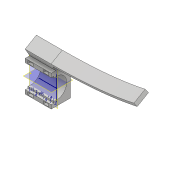
# Autodesk Inventor part: abrazadera_leds
Saved by Autodesk Inventor 2018 (Build 220112000, 112)
## iProperties
Created: 2018-08-01
Part Number: abrazadera_leds
Material: Generic
Document SubType Name: Sheet Metal
Designer: Bardo91
Density: 1 g/cm^3
Sheet Metal Rule: Default_mm
Appearance: Default
Author: Bardo91
Autodesk Inventor part; units mm, degrees
ref_plane "YZ Plane" through (0, 0, 0) normal (1, 0, 0) x (0, 1, 0)
ref_plane "XZ Plane" through (0, 0, 0) normal (0, 1, 0) x (-1, 0, 0)
ref_plane "XY Plane" through (0, 0, 0) normal (0, 0, 1) x (1, 0, 0)
sketch "Sketch1" plane through (0, 0, 0) normal (1, 0, 0) x (0, 1, 0)
  arc A0 (-2, -7.746) -> (-2, 7.746) centre (0, 0) ccw
  line L0 (0, 0) -> (-2, 0)
  line L1 (-2, 7.746) -> (-2, 9)
  line L2 (-2, 9) -> (-4, 9)
  line L3 (-4, 9) -> (-4, 12)
  line L4 (-4, 12) -> (11, 12)
  line L5 (-2, 0) -> (-2, -9)
  line L6 (-2, -9) -> (-4, -9)
  line L7 (-4, -9) -> (-4, -12)
  line L8 (-4, -12) -> (11, -12)
  line L9 (11, -12) -> (11, 12)
  line L10 (11, 12) -> (6, 20.6603)
  line L11 (11, 12) -> (21, 12) construction
  line L12 (6, 20.6603) -> (-2.6603, 15.6603)
  line L13 (-2.6603, 15.6603) -> (-0.547, 12)
  dimension "d0" = 16
  dimension "d1" = 2
  dimension "d2" = 9
  dimension "d3" = 2
  dimension "d4" = 3
  dimension "d5" = 15
  dimension "d6" = 9
  dimension "d7" = 3
  dimension "d8" = 10
  dimension "d9" = 120
  dimension "d10" = 10
  constraints: 28 end point, 9 perpendicular, 3 horizontal, 2 point on circle, 2 point on line, 1 centre point, 1 coincident, 1 equal length, 1 vertical
  measures "d0" diameter of A0
  measures "d1" distance of L0.start L0.end
  measures "d2" distance of L0.end L1.end
  measures "d3" distance of L1.end L2.end
  measures "d4" distance of L2.end L3.end
  measures "d5" distance of L3.end L4.end
  measures "d6" distance of L0.end L5.end
  measures "d7" distance of L6.end L7.end
  measures "d8" distance of L4.end L10.end
  measures "d9" angle of L11 L10
  measures "d10" distance of L10.end L12.end
extrude "Extrusion1" add sketch "Sketch1" along normal blind 20
ref_plane "Work Plane1" through (20, 8, 0) normal (0, 0, -1) x (-1, 0, 0)
ref_plane "Work Plane2" through (0, 0, 12) normal (0, 1, 0) x (1, 0, 0)
sketch "Sketch3" plane through (0, 0, 12) normal (0, 1, 0) x (1, 0, 0)
  line L0 (0, 21) -> (20, 21) projected
  line L1 (10, 21) -> (10, 22.5)
  line L2 (10, 22.5) -> (14, 22.5)
  line L3 (14, 22.5) -> (14, 21.5)
  line L4 (14, 21.5) -> (18, 21.5)
  line L5 (18, 21.5) -> (18, 23.5)
  line L6 (18, 23.5) -> (14, 23.5)
  line L7 (14, 23.5) -> (14, 22.5)
  line L8 (10, 22.5) -> (6, 22.5)
  line L9 (6, 22.5) -> (6, 23.5)
  line L10 (6, 23.5) -> (2, 23.5)
  line L11 (2, 23.5) -> (2, 21.5)
  line L12 (2, 21.5) -> (6, 21.5)
  line L13 (6, 22.5) -> (6, 21.5)
  line L14 (0, 3) -> (20, 3) projected
  line L15 (20, 21) -> (20, 3)
  line L16 (20, 20) -> (20, 4) projected
  line L17 (20, 12) -> (6.2446, 12)
  line L18 (0, 3) -> (20, 3)
  line L19 (10, 3) -> (10, 1.5)
  line L20 (10, 1.5) -> (14, 1.5)
  line L21 (14, 1.5) -> (14, 2.5)
  line L22 (14, 2.5) -> (18, 2.5)
  line L23 (18, 2.5) -> (18, 0.5)
  line L24 (18, 0.5) -> (14, 0.5)
  line L25 (14, 0.5) -> (14, 1.5)
  line L26 (10, 1.5) -> (6, 1.5)
  line L27 (6, 1.5) -> (6, 0.5)
  line L28 (6, 0.5) -> (2, 0.5)
  line L29 (2, 0.5) -> (2, 2.5)
  line L30 (2, 2.5) -> (6, 2.5)
  line L31 (6, 1.5) -> (6, 2.5)
  point P0 (0, 12)
  point P1 (20, 4.254)
  point P2 (20, 19.746)
  dimension "d25" = 1.5
  dimension "d26" = 4
  dimension "d27" = 1
  dimension "d28" = 4
  dimension "d29" = 2
  dimension "d30" = 4
  dimension "d31" = 1
  dimension "d32" = 4
  dimension "d33" = 2
  constraints: 58 end point, 14 point on line, 12 symmetric about line, 6 perpendicular, 2 horizontal, 2 midpoint, 1 vertical
  measures "d25" distance of L1.start L1.end
  measures "d26" distance of L1.end L2.end
  measures "d27" distance of L2.end L3.end
  measures "d28" distance of L3.end L4.end
  measures "d29" distance of L4.end L5.end
  measures "d30" distance of L1.end L8.end
  measures "d31" distance of L8.end L9.end
  measures "d32" distance of L9.end L10.end
  measures "d33" distance of L10.end L11.end
revolve "Revolution1" cut sketch "Sketch3" angle 180 about axis through (20, 0, 0) along (1, 0, 0) contours L13 L12 L11 L10 L9 | L7 L6 L5 L4 L3
extrude "Extrusion3" cut sketch "Sketch3" against normal blind 20
sketch "Sketch5" plane through (0, 6, 20.6603) normal (0, 0.866, 0.5) x (1, 0, 0)
  line L0 (0, 10) -> (0, 0) projected
  line L1 (0, 0) -> (20, 0) projected
  line L2 (0, 0) -> (20, 0)
  arc A0 (93.2847, -16.3126) -> (20, 0) centre (20, -172.7725) ccw
  arc A1 (92.0249, -19.0024) -> (20, -2.9702) centre (20, -172.7725) ccw
  line L3 (20, -2.9702) -> (0, -2.9702)
  line L4 (0, 0) -> (0, -2.9702)
  line L5 (93.2847, -16.3126) -> (92.0249, -19.0024)
  point P0 (0, 14.8923)
  constraints: 8 end point, 4 point on circle, 2 centre point, 1 horizontal, 1 perpendicular, 1 tangent, 1 other
extrude "Extrusion4" add sketch "Sketch5" against normal up to surface (10 mm away)
equation "\"BendRadius\" = Thickness"
equation "\"BendReliefWidth\" = Thickness"
equation "\"BendReliefDepth\" = 0.5 * Thickness"
equation "\"CornerReliefSize\" = 4 * Thickness"
equation "\"MinimumRemnant\" = 2 * Thickness"
equation "\"TransitionRadius\" = BendRadius"
equation "\"JacobiRadiusSize\" = BendRadius"
equation "\"GapSize\" = Thickness"
equation "\"Thickness\" = 0.5"
body "Solid1"
